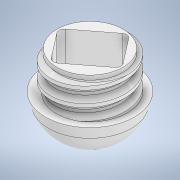
# Autodesk Inventor part: SmartEgg Shell
Saved by Autodesk Inventor 2020 (Build 240168000, 168)
## iProperties
Created: 2019-11-26
Part Number: SmartEgg Shell
Material: Generic
Document SubType Name: Modeling
Designer: Andrew
Density: 1 g/cm^3
Appearance: White
d0: 1.000 ul
d17: 1.000 ul
d18: 25.000 mm
d19: 50.000 mm
d20: 1.000 mm
d21: 17.000 mm
d22: 5.000 mm
d23: 2.000 mm
d24: 12.500 mm
d25: 0.250 mm
d26: 20.000 mm
d27: 3.000 mm
d28: 1.500 mm
d30: 1.000 mm
d32: 0.500 mm
d33: 0.500 mm
d35: 45.00 deg
d36: 0.250 mm
d37: 2.000 mm
d38: 2.000 mm
d41: 8.708 mm
d43: 3.000 ul
d44: 0.00 deg
d50: 8.708 mm
d52: 1.000 ul
d53: 0.00 deg
d61: 2.500 mm
d29: 69.904 mm
d39: 7.000 mm
Thread_Pitch: 4.354 mm
BATT_Width: 24.750 mm
PCB_Width: 22.850 mm
Author: Andrew
Autodesk Inventor part; units mm, degrees
ref_plane "YZ Plane" through (0, 0, 0) normal (1, 0, 0) x (0, 1, 0)
ref_plane "XZ Plane" through (0, 0, 0) normal (0, 1, 0) x (-1, 0, 0)
ref_plane "XY Plane" through (0, 0, 0) normal (0, 0, 1) x (1, 0, 0)
derived "SmartEgg Housing Main.ipt"
sketch "Sketch3" plane through (0, 0, 0) normal (0, 0, 1) x (1, 0, 0)
  line L0 (25.5, 9.75) -> (25.5, -9.25)
  line L1 (26.5, 12) -> (26.5, -11.5)
  line L2 (-26.5, -11.5) -> (-26.5, 12)
  line L3 (-7.4558, 6.9665) -> (-15.25, -6.5335)
  line L4 (-15.5, -6.4665) -> (-7.7058, 7.0335)
  line L5 (-26.5, 12) -> (-7.7058, 12)
  line L6 (-7.4558, 12) -> (26.5, 12)
  line L7 (-25.5, 9.75) -> (7.2942, 9.75)
  line L8 (7.5442, 9.75) -> (25.5, 9.75)
  line L9 (25.5, -9.25) -> (-0.25, -9.25)
  line L10 (-0.5, -9.25) -> (-25.5, -9.25)
  line L11 (26.5, -11.5) -> (-15.25, -11.5)
  line L12 (-15.5, -11.5) -> (-26.5, -11.5)
  line L13 (25.5, 0) -> (25.5, -1.75) construction
  line L14 (-25.5, -1.75) -> (-25.5, 0) construction
  line L15 (-25.5, -3.25) -> (-0.5, -3.25)
  line L16 (-0.5, -3.25) -> (-0.5, -4.25)
  line L17 (-0.5, -4.25) -> (-25.5, -4.25)
  line L18 (-25.5, -9.25) -> (-25.5, -4.25)
  line L19 (-25.5, -3.25) -> (-25.5, 9.75)
  line L20 (-7.5808, 12) -> (-7.5808, 7) construction
  line L21 (-7.5808, 7) -> (-15.375, -6.5) construction
  line L22 (-15.375, -6.5) -> (-15.375, -11.5) construction
  line L23 (-7.7058, 12) -> (-7.7058, 10.75)
  line L24 (-7.7058, 10.75) -> (7.2942, 10.75)
  line L25 (7.2942, 10.75) -> (7.2942, 9.75)
  line L26 (7.5442, 9.75) -> (7.5442, 11)
  line L27 (7.5442, 11) -> (-7.4558, 11)
  line L28 (-7.4558, 11) -> (-7.4558, 12)
  line L29 (-15.5, -11.5) -> (-15.5, -10.25)
  line L30 (-15.5, -10.25) -> (-0.5, -10.25)
  line L31 (-0.5, -10.25) -> (-0.5, -9.25)
  line L32 (-0.25, -9.25) -> (-0.25, -10.5)
  line L33 (-0.25, -10.5) -> (-15.25, -10.5)
  line L34 (-15.25, -10.5) -> (-15.25, -11.5)
  line L35 (-7.7058, 10.75) -> (-7.7058, 7.0335)
  line L36 (-7.4558, 6.9665) -> (-7.4558, 11)
  line L37 (-15.5, -10.25) -> (-15.5, -6.4665)
  line L38 (-15.25, -6.5335) -> (-15.25, -10.5)
  line L39 (7.2942, 9.75) -> (7.2942, 7.0335)
  line L40 (7.2942, 7.0335) -> (-0.5, -6.4665)
  line L41 (-0.5, -6.4665) -> (-0.5, -9.25)
  line L42 (-0.25, -9.25) -> (-0.25, -6.5335)
  line L43 (-0.25, -6.5335) -> (7.5442, 6.9665)
  line L44 (7.5442, 6.9665) -> (7.5442, 9.75)
  line L45 (-0.375, -11.5) -> (-0.375, -6.5) construction
  line L46 (-0.375, -6.5) -> (7.4192, 7) construction
  line L47 (7.4192, 7) -> (7.4192, 12) construction
  line L48 (11.5, -9.25) -> (16.5, -9.25)
  line L49 (16.5, -9.25) -> (14, -6.75)
  line L50 (14, -6.75) -> (11.5, -6.75)
  line L51 (11.5, -6.75) -> (11.5, -9.25)
  point P0 (0, 0)
derived "SmartEgg Housing Cap.ipt"
sketch "Housing Largest Area" plane through (0, -10.3291, -13.7529) normal (0, 0.792624, -0.6097108) x (0, 0.6097108, 0.792624)
  line L0 (30.2021, 26.5) -> (29.0299, 26.5)
  line L1 (17.3511, 26.5) -> (17.3511, -26.5)
  line L2 (17.3511, -26.5) -> (34.7021, -26.5)
  line L3 (34.7021, -26.5) -> (34.7021, 22)
  line L4 (10.187, -26.5) -> (24.5152, -26.5) construction
  line L5 (24.5152, 26.5) -> (10.187, 26.5) construction
  line L6 (11.6106, 20.5) -> (9.9705, 20.5) construction
  line L7 (9.9705, 20.5) -> (9.9705, 24.5) construction
  ellipse E0 centre (8.3304, 24.5) end of major axis (9.9705, 24.5) minor radius 1 (9.9705, 24.5) -> (8.3304, 25.5) ccw construction
  line L8 (8.3304, 25.5) -> (2.1723, 25.5) construction
  line L9 (2.1723, 25.5) -> (2.1723, -0.25) construction
  line L10 (2.1723, -0.25) -> (1, -0.25) construction
  line L11 (1, -0.25) -> (1, -15.25) construction
  line L12 (1, -15.25) -> (0, -15.25) construction
  line L13 (0, -15.25) -> (0, 24.5) construction
  arc A0 (2, 26.5) -> (0, 24.5) centre (2, 24.5) ccw construction
  line L14 (2, 26.5) -> (16.941, 26.5) construction
  line L15 (16.941, 26.5) -> (16.941, 25.5) construction
  line L16 (16.941, 25.5) -> (14.0708, 25.5) construction
  line L17 (14.0708, 25.5) -> (14.0708, 22.4142) construction
  ellipse E1 centre (12.4307, 22.4142) end of major axis (14.0708, 22.4142) minor radius 1 (13.5904, 21.7071) -> (14.0708, 22.4142) ccw construction
  line L18 (13.5904, 21.7071) -> (11.6106, 20.5) construction
  arc A1 (34.7021, 24.5) -> (32.7021, 26.5) centre (32.7021, 24.5) ccw construction
  line L19 (34.7021, 24.5) -> (34.7021, -7.4558) construction
  line L20 (34.7021, -7.4558) -> (33.7021, -7.4558) construction
  line L21 (33.7021, -7.4558) -> (33.7021, 7.5442) construction
  line L22 (33.7021, 7.5442) -> (32.5299, 7.5442) construction
  line L23 (32.5299, 7.5442) -> (32.5299, 25.5) construction
  line L24 (32.5299, 25.5) -> (21.0413, 25.5) construction
  line L25 (21.0413, 25.5) -> (21.0413, 26.5) construction
  line L26 (21.0413, 26.5) -> (32.7021, 26.5) construction
  arc A2 (34.7021, 22) -> (30.2021, 26.5) centre (30.2021, 22) ccw
  arc A3 (32.5299, 22) -> (29.0299, 25.5) centre (29.0299, 22) ccw
  line L27 (32.5299, 22) -> (34.7021, 22)
  line L28 (29.0299, 25.5) -> (29.0299, 26.5)
  line L29 (29.0299, 26.5) -> (17.3511, 26.5)
  point P0 (17.1986, 0)
  point P1 (17.3511, 0)
sketch "ESP32 Feather" plane through (0, 0, 0) normal (0, 0, 1) x (1, 0, 0)
  line L0 (-25.5, 0) -> (25.5, 0)
  line L1 (25.5, 0) -> (25.5, -1.75)
  line L2 (25.5, -1.75) -> (-25.5, -1.75)
  line L3 (-25.5, -1.75) -> (-25.5, 0)
  line L4 (0, 0) -> (-25.5, 0)
  line L5 (-25.5, 0) -> (-25.5, 0.8)
  line L6 (-25.5, 0.8) -> (0, 0.8)
  line L7 (0, 0.8) -> (0, 0)
  line L8 (-0.9, 0.8) -> (-18.55, 0.8)
  line L9 (-18.55, 0.8) -> (-18.55, 3.15)
  line L10 (-18.55, 3.15) -> (-0.9, 3.15)
  line L11 (-0.9, 3.15) -> (-0.9, 0.8)
  line L12 (10.75, 0) -> (18.75, 0)
  line L13 (18.75, 0) -> (18.75, 5.5)
  line L14 (18.75, 5.5) -> (10.75, 5.5)
  line L15 (10.75, 5.5) -> (10.75, 0)
  line L16 (25.6, 0) -> (19.95, 0)
  line L17 (19.95, 0) -> (19.95, 2.5)
  line L18 (19.95, 2.5) -> (25.6, 2.5)
  line L19 (25.6, 2.5) -> (25.6, 0)
  point P0 (0, 0)
  point P1 (0, 0)
  point P2 (19.95, 0)
sketch "Shell Sketch" plane through (0, -10.3291, -13.7529) normal (0, 0.792624, -0.6097108) x (0, 0.6097108, 0.792624)
  arc A0 (40.9669, -18.122) -> (29.5168, 33.2086) centre (-6.2647, -1.7154) ccw
  arc A1 (17.3511, -34.9187) -> (29.8511, -31.5693) centre (17.3511, -9.9187) ccw construction
  line L0 (17.3511, -34.9187) -> (17.3511, -31.5693) construction
  line L1 (17.3511, 9.75) -> (36.2021, 9.75)
  line L2 (17.3511, 26.5) -> (17.3511, -26.5) construction
  line L3 (34.7021, -26.5) -> (35.4251, -27.1909) construction
  arc A2 (29.5168, 33.2086) -> (17.3511, 38.3345) centre (17.3511, 21.3345) ccw
  line L4 (17.3511, 38.3345) -> (17.3511, 35.4766)
  line L5 (17.3511, 35.4766) -> (22.3511, 35.4766)
  arc A3 (28.0855, 31.8117) -> (22.3511, 35.4766) centre (17.3511, 21.3345) ccw
  arc A4 (37.2672, 18.5076) -> (28.0855, 31.8117) centre (-6.2647, -1.7154) ccw
  arc A5 (34.7021, 22) -> (30.2021, 26.5) centre (30.2021, 22) ccw construction
  line L6 (36.2021, 9.75) -> (36.2021, -11.5693)
  line L7 (36.2021, -11.5693) -> (42.7547, -11.5693)
  line L8 (39.2021, 9.75) -> (39.2021, -11.3193)
  line L9 (39.2021, -11.3193) -> (42.8042, -11.3193)
  line L10 (17.3511, -31.5693) -> (29.8511, -31.5693)
  arc A6 (29.8511, -31.5693) -> (40.9669, -18.122) centre (17.3511, -9.9187) ccw
  line L11 (17.3511, -31.5693) -> (17.3511, 9.75)
  line L12 (34.7021, -26.5) -> (34.7021, 22) construction
  line L13 (20.552, 10.75) -> (17.1986, 10.75) construction
  arc A7 (39.2021, 9.75) -> (37.2672, 18.5076) centre (18.4156, 9.75) ccw
  point P0 (17.1986, 0)
  point P1 (39.2021, 13.6718)
  dimension "d18" = 25
  dimension "d19" = 50
  dimension "d20" = 1
  dimension "d21" = 17
  dimension "d22" = 5
  dimension "d23" = 2
  dimension "d24" = 12.5
  dimension "d25" = 0.25
  dimension "d26" = 20
  dimension "d27" = 3
  dimension "d28" = 1.5
  dimension "d29" = 69.9038
  dimension "d30" = 1
  constraints: 22 end point, 19 point on circle, 7 centre point, 7 line through centre, 6 perpendicular, 6 tangent, 4 collinear, 4 vertical, 2 concentric, 2 point on line, 1 coincident, 1 horizontal
  measures "d18" radius of A1
  measures "d19" radius of A0
  measures "d20" distance of L3.start L3.end
  measures "d21" radius of A2
  measures "d22" distance of L4.end L5.end
  measures "d23" radial gap between concentric circles of A0 A4
  measures "d24" distance of L0.end L10.end
  measures "d25" distance between parallel lines of L7 L9
  measures "d26" distance between parallel lines of L10 L7
  measures "d27" distance between parallel lines of L8 L6
  measures "d28" distance between parallel lines of L12 L6
  measures "d29" distance from line of L10 L4.start
  measures "d30" distance between parallel lines of L1 L13
sketch "Thread Sketch" plane through (0, -10.3291, -13.7529) normal (0, 0.792624, -0.6097108) x (0, 0.6097108, 0.792624)
  line L0 (36.2021, 9.75) -> (36.2021, -11.5693) construction
  line L1 (39.2021, 9.75) -> (39.2021, -11.3193) construction
  line L2 (36.2021, 9.75) -> (38.7021, 7.25)
  line L3 (38.7021, 7.25) -> (38.7021, 5.25)
  line L4 (38.7021, 5.25) -> (36.2021, 2.75)
  line L5 (36.2021, 2.75) -> (36.2021, 9.75)
  line L6 (39.2021, 5.3964) -> (36.7021, 2.8964)
  line L7 (36.7021, 2.8964) -> (36.7021, 0.8964)
  line L8 (36.7021, 0.8964) -> (39.2021, -1.6036)
  line L9 (39.2021, -1.6036) -> (39.2021, 5.3964)
  line L10 (38.7021, 6.25) -> (36.2021, 6.25) construction
  line L11 (36.7021, 1.8964) -> (39.2021, 1.8964) construction
  point P0 (17.1986, 0)
  dimension "d32" = 0.5
  dimension "d33" = 0.5
  dimension "d35" = 45
  dimension "d36" = 0.25
  dimension "d37" = 2
  dimension "d38" = 2
  dimension "d39" = 7
  dimension "Thread_Pitch" = 4.354
  constraints: 20 end point, 4 midpoint, 3 parallel, 2 horizontal, 2 point on line, 2 other
  measures "d32" distance between parallel lines of L1 L3
  measures "d33" distance between parallel lines of L0 L7
  measures "d35" angle of L0 L4
  measures "d36" distance between parallel lines of L6 L4
  measures "d37" distance of L2.end L3.end
  measures "d38" distance of L6.end L7.end
  measures "d39" distance of L4.end L0.start
revolve "Revolution1" add sketch "Shell Sketch" angle 360 about axis through (-31.5693, 0.25, 0) along (1, 0, 0) contours A6 L10 L11 L1 L6 L7 A0
coil "Coil1" sketch "Thread Sketch" operation add axis through (-31.5693, 0.25, 0) along (-1, 0, 0) pitch 8.708 turns 3 hand right separate body contours L2 L3 L4 L5
coil "Coil2" sketch "Thread Sketch" operation add axis through (-31.5693, 0.25, 0) along (1, 0, 0) pitch 8.708 turns 1 hand right bodies 2 contours L2 L3 L4 L5
sketch "Thread Mask" plane through (0, -10.3291, -13.7529) normal (0, 0.792624, -0.6097108) x (0, 0.6097108, 0.792624)
  line L0 (39.2021, 7.25) -> (36.2021, 7.25)
  line L1 (36.2021, 7.25) -> (36.2021, -11.5693)
  line L2 (36.2021, -11.5693) -> (39.2021, -11.5693)
  line L3 (39.2021, -11.5693) -> (39.2021, 7.25)
  line L4 (36.2021, 9.75) -> (36.2021, -11.5693) construction
  line L5 (39.2021, 9.75) -> (39.2021, -11.3193) construction
  point P0 (17.1986, 0)
  dimension "d61" = 2.5
  constraints: 8 end point, 2 parallel, 1 collinear, 1 horizontal, 1 perpendicular
  measures "d61" distance from line of L4.start L0
revolve "Revolution4" cut sketch "Thread Mask" angle 360 about axis through (-31.5693, 0.25, 0) along (1, 0, 0) keep common part bodies 2
combine bodies "Combine1" operation type add bodies to combine 1 2
sketch "Sketch10" plane through (9.75, 0.25, 0) normal (1, 0, 0) x (0, 0, -1)
  line L0 (-11.625, -12) -> (11.625, -12)
  line L1 (14.625, -9) -> (14.625, 9)
  line L2 (11.625, 12) -> (-11.625, 12)
  line L3 (-14.625, 9) -> (-14.625, -9)
  line L4 (-14.625, 0) -> (14.625, 0) construction
  arc A0 (-11.625, 12) -> (-14.625, 9) centre (-11.625, 9) ccw
  arc A1 (14.625, 9) -> (11.625, 12) centre (11.625, 9) ccw
  arc A2 (11.625, -12) -> (14.625, -9) centre (11.625, -9) ccw
  arc A3 (-14.625, -9) -> (-11.625, -12) centre (-11.625, -9) ccw
  point P0 (0, -0.25)
  point P1 (14.625, 12)
  point P2 (-14.625, 12)
  point P3 (0, -11.75)
  point P4 (0, -11.75)
  point P5 (0, -11.75)
  point P6 (0, 11.75)
  point P7 (0, 11.75)
  point P8 (0, 11.75)
  point P9 (0, 0)
  point P10 (0, 0)
  point P11 (0, 0)
  point P12 (0, 0)
  dimension "d64" = 0.25
  dimension "d65" = 29.25
  dimension "d66" = 3
  constraints: 10 end point, 8 point on circle, 8 tangent, 4 centre point, 4 point on line, 3 equal radius, 3 midpoint, 2 parallel, 1 coincident, 1 horizontal, 1 perpendicular
  measures "d64" distance from line of L0 point (0, -11.75)
  measures "d65" distance of point (14.625, 12) point (-14.625, 12)
  measures "d66" radius of A0
sketch "Sketch11" plane through (0, 0, 0) normal (0, 0, 1) x (1, 0, 0)
  line L0 (9.75, 19.1011) -> (9.75, -18.6011) projected
  line L1 (9.75, 0.25) -> (-26.5, 0.25)
  line L2 (-26.5, -11.5) -> (-26.5, 12) construction
  point P0 (0, 0)
  dimension "d67" = 36.25
  constraints: 2 end point, 2 midpoint, 1 horizontal
  measures "d67" distance of L1.start L1.end
extrude "Extrusion1" cut sketch "Sketch10" against normal blind 36.25 bodies 1
fillet "Fillet1" radius 2.25 8 edges at (-26.5, 11.3713, 13.7463) (-26.5, 12.25, 0) (-26.5, 11.3713, -13.7463) (-26.5, 0.25, -14.625) (-26.5, -10.8713, -13.7463) (-26.5, -11.75, 0) (-26.5, -10.8713, 13.7463) (-26.5, 0.25, 14.625)
ref_plane "Work Plane2" through (0, -10.3291, -13.7529) normal (0, 0.792624, -0.6097108) x (0, 0.6097108, 0.792624)
equation "\"d38\" = d37"
equation "\"d41\" = 2 * Thread_Pitch"
equation "\"d50\" = 2 * Thread_Pitch"
equation "\"d68\" = d67"
body "Solid1"
body "Solid3"
